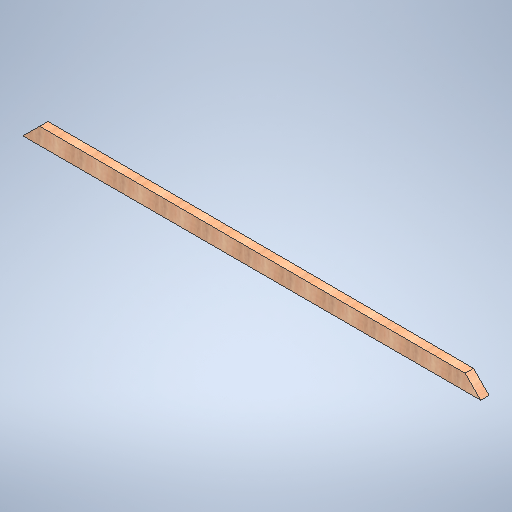
# Autodesk Inventor part: 2x4xidk
Saved by Autodesk Inventor 2025 (Build 290162000, 162)
## iProperties
Created: 2024-08-19
Part Number: 2x4xidk
Material: Generic
Document SubType Name: Modeling
Designer: Cupri
Density: 1 g/cm^3
Appearance: Default
Author: Cupri
Autodesk Inventor part; units mm, degrees
ref_plane "YZ Plane" through (0, 0, 0) normal (1, 0, 0) x (0, 1, 0)
ref_plane "XZ Plane" through (0, 0, 0) normal (0, 1, 0) x (-1, 0, 0)
ref_plane "XY Plane" through (0, 0, 0) normal (0, 0, 1) x (1, 0, 0)
sketch "Sketch1" plane through (0, 0, 0) normal (0, 0, 1) x (1, 0, 0)
  line L0 (-1301.355, 12.893) -> (1280.7246, 6.3845)
  line L1 (-1301.6111, -88.7066) -> (-1402.6998, -88.4518)
  line L2 (-1301.355, 12.893) -> (-1402.6998, -88.4518)
  line L3 (-1402.6998, -88.4518) -> (1375.5609, -88.4518)
  line L4 (1280.7246, 6.3845) -> (1375.5609, -88.4518)
  point P0 (0, 0)
  dimension "d0" = 101.6
  constraints: 10 end point, 1 horizontal
  measures "d0" distance of L0.start L1.start
extrude "Extrusion1" add sketch "Sketch1" along normal blind 50.8
body "Solid1"
